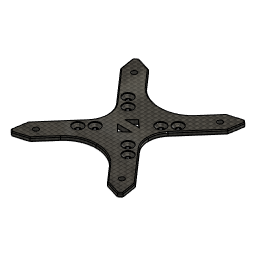
middle_plate (Autodesk Fusion 360 design; units mm, degrees)
Autodesk Fusion 360 part; units mm, degrees
sketch "Sketch1" plane through (0, 0, 0) normal (0, 1, 0) x (1, 0, 0)
  line L0 (25.882765, 29.580303) -> (21.367305, 33.53133) construction
  line L1 (25.882765, 29.580303) -> (30.398225, 25.629275) construction
  line L2 (23.572116, 36.051114) -> (14.916845, 26.159376)
  arc A0 (0, 19.5) -> (14.916845, 26.159376) centre (0.237925, 39.003431) ccw
  line L3 (34.026215, 36.985626) -> (33.083891, 37.81016)
  circle A1 centre (10, 10) radius 1.015
  line L4 (-15, 15) -> (15, 15) construction
  line L5 (-21.367305, 33.53133) -> (7.972627, -0.000021) construction
  line L6 (30.398225, 25.629275) -> (7.972612, 0.000001) construction
  arc A2 (-14.916845, 26.159376) -> (0, 19.5) centre (-0.237925, 39.003431) ccw
  line L7 (21.367305, 33.53133) -> (-7.972627, -0.000021) construction
  line L8 (32.141566, 38.634694) -> (33.083891, 37.81016)
  line L9 (23.572116, 36.051114) -> (32.141566, 38.634694)
  line L10 (-32.141566, 38.634694) -> (-33.083891, 37.81016)
  line L11 (32.603036, 28.149059) -> (34.026215, 36.985626)
  line L12 (0, 0) -> (0, 40.717058) construction
  line L13 (-32.603036, 28.149059) -> (-34.026215, 36.985626)
  line L14 (-10, 10) -> (10, 10) construction
  line L15 (-25.882765, 29.580303) -> (-21.367305, 33.53133) construction
  line L16 (-23.572116, 36.051114) -> (-32.141566, 38.634694)
  line L17 (-23.572116, 36.051114) -> (-14.916845, 26.159376)
  line L18 (-34.026215, 36.985626) -> (-33.083891, 37.81016)
  line L19 (-25.882765, 29.580303) -> (-30.398225, 25.629275) construction
  circle A3 centre (-10, 10) radius 1.015
  line L20 (-0.000752, 6.361835) -> (-4.075325, 2.287262)
  line L21 (4.583143, 2.287262) -> (-0.000752, 6.361835)
  line L22 (0, 0) -> (-12.395289, 0.000003)
  line L23 (-4.075325, 2.287262) -> (4.583143, 2.287262)
  line L24 (-32.603036, 28.149059) -> (-15.606858, 8.724856)
  arc A4 (-12.395289, 0.000003) -> (-15.606858, 8.724856) centre (-25.378902, 0.174315) ccw
  line L25 (32.603036, 28.149059) -> (15.606858, 8.724856)
  arc A5 (15.606858, 8.724856) -> (12.395289, 0.000003) centre (25.378902, 0.174315) ccw
  line L26 (0, 0) -> (50.000001, 0) construction
  arc A6 (0, -19.5) -> (-14.916845, -26.159376) centre (-0.237925, -39.003431) ccw
  line L27 (-15, -15) -> (15, -15) construction
  line L28 (30.398225, -25.629275) -> (7.972612, -0.000001) construction
  line L29 (-32.603036, -28.149059) -> (-15.606858, -8.724856)
  line L30 (32.603036, -28.149059) -> (15.606858, -8.724856)
  arc A7 (12.395289, -0.000003) -> (15.606858, -8.724856) centre (25.378902, -0.174315) ccw
  line L31 (21.367305, -33.53133) -> (-7.972627, 0.000021) construction
  line L32 (-23.572116, -36.051114) -> (-32.141566, -38.634694)
  line L33 (0, 0) -> (-12.395289, -0.000003)
  line L34 (-32.603036, -28.149059) -> (-34.026215, -36.985626)
  circle A8 centre (-10, -10) radius 1.015
  line L35 (-0.000752, -6.361835) -> (-4.075325, -2.287262)
  line L36 (23.572116, -36.051114) -> (14.916845, -26.159376)
  circle A9 centre (10, -10) radius 1.015
  line L37 (-25.882765, -29.580303) -> (-30.398225, -25.629275) construction
  arc A10 (-15.606858, -8.724856) -> (-12.395289, -0.000003) centre (-25.378902, -0.174315) ccw
  line L38 (-21.367305, -33.53133) -> (7.972627, 0.000021) construction
  line L39 (4.583143, -2.287262) -> (-0.000752, -6.361835)
  line L40 (-4.075325, -2.287262) -> (4.583143, -2.287262)
  line L41 (25.882765, -29.580303) -> (21.367305, -33.53133) construction
  line L42 (25.882765, -29.580303) -> (30.398225, -25.629275) construction
  line L43 (-34.026215, -36.985626) -> (-33.083891, -37.81016)
  line L44 (-23.572116, -36.051114) -> (-14.916845, -26.159376)
  line L45 (23.572116, -36.051114) -> (32.141566, -38.634694)
  line L46 (34.026215, -36.985626) -> (33.083891, -37.81016)
  line L47 (32.603036, -28.149059) -> (34.026215, -36.985626)
  line L48 (0, 0) -> (0, -40.717058) construction
  arc A11 (14.916845, -26.159376) -> (0, -19.5) centre (0.237925, -39.003431) ccw
  line L49 (-25.882765, -29.580303) -> (-21.367305, -33.53133) construction
  line L50 (32.141566, -38.634694) -> (33.083891, -37.81016)
  line L51 (-32.141566, -38.634694) -> (-33.083891, -37.81016)
  line L52 (-10, -10) -> (10, -10) construction
  circle A12 centre (-26.106671, -29.832074) radius 1.525
  circle A13 centre (-19.710816, -22.523297) radius 1.525
  line L53 (-25.88455, -29.578249) -> (-30.399804, -25.626985) construction
  line L54 (-25.88455, -29.578249) -> (-21.369297, -33.529512) construction
  circle A14 centre (-19.710816, 22.523297) radius 1.525
  circle A15 centre (-26.106671, 29.832074) radius 1.525
  circle A16 centre (19.710816, 22.523297) radius 1.525
  circle A17 centre (26.106671, 29.832074) radius 1.525
  circle A18 centre (19.710816, -22.523297) radius 1.525
  circle A19 centre (26.106671, -29.832074) radius 1.525
  circle A20 centre (0, 0) radius 6.361835
  line L55 (15.25, 15.25) -> (-15.25, 15.25) construction
  line L56 (-15.25, 15.25) -> (-15.25, -15.25) construction
  line L57 (-15.25, -15.25) -> (15.25, -15.25) construction
  line L58 (15.25, -15.25) -> (15.25, 15.25) construction
  line L59 (15.25, 15.25) -> (-15.25, -15.25) construction
  line L60 (-15.25, 15.25) -> (15.25, -15.25) construction
  circle A21 centre (15.25, 15.25) radius 1.525
  circle A22 centre (-15.25, 15.25) radius 1.525
  circle A23 centre (-15.25, -15.25) radius 1.525
  circle A24 centre (15.25, -15.25) radius 1.525
  point P0 (15, 15)
  point P1 (10, 10)
  point P2 (0, 17.5)
  point P3 (0, 40.717058)
  point P4 (-7.972609, 0)
  point P5 (7.972609, 0)
  point P6 (-7.972609, 0)
  point P7 (7.972609, 0)
  point P8 (0, -40.717058)
  point P9 (-7.972609, 0)
  point P10 (-7.972609, 0)
  point P11 (0, -17.5)
  point P12 (7.972609, 0)
  point P13 (7.972609, 0)
  point P14 (10, -10)
  point P15 (15, -15)
  point P16 (15.25, 15.25)
  dimension "d3" = 30
  dimension "d5" = 20
  dimension "d42" = 2.03
  dimension "d90" = 6
  dimension "d91" = 6
  dimension "d75" = 30.5
  dimension "d76" = 30.5
  dimension "d77" = 3.05
  dimension "d78" = 3.05
  dimension "d79" = 3.05
  dimension "d80" = 3.05
  constraint coincident L12.start L22.start
  constraint coincident L14.start A3.centre
  constraint perpendicular L5 L15
  constraint symmetric L22.start L26.start L12
  constraint tangent L5 A2
  constraint coincident A0.start L12
  constraint symmetric A0.start A2.end L12
  constraint symmetric A0 A2 L12
  constraint symmetric L12 A4 A5
  constraint perpendicular L12 L26
  constraint symmetric L12.start L26 L22.start
  constraint symmetric P0 L26 P15
  constraint symmetric P1 L26 P14
  constraint symmetric P2 L26 P11
  constraint symmetric A0.start L26 A6.start
  constraint symmetric L4.start L26 L27.start
  constraint symmetric L14.start L26 A8.centre
  constraint symmetric A0 L26 A11
  constraint symmetric A1 L26 A9
  constraint symmetric A2 L26 A6
  constraint symmetric A3 L26 A8
  constraint symmetric A4 L26 A10
  constraint symmetric A5 L26 A7
  constraint symmetric L26 A12 A15
  constraint symmetric L26 A13 A14
  constraint symmetric L12 A12 A19
  constraint symmetric L12 A13 A18
  constraint symmetric L12 A14 A16
  constraint symmetric L12 A15 A17
  constraint horizontal L55
  constraint perpendicular L55 L56
  constraint parallel L55 L57
  constraint parallel L56 L58
  constraint coincident L59 L12.start
  constraint coincident L60 L12.start
  constraint coincident P16 L55.start
  constraint coincident L55.end L56.start
  constraint coincident L56.end L57.start
  constraint coincident L57.end L58.start
  measures "d3" distance of P0 L4.start
  measures "d5" distance of P1 L14.start
  measures "d42" diameter of A3
  measures "d75" distance of L56.end L57.end
  measures "d76" distance of L55.end L56.end
  measures "d77" diameter of A21
  measures "d78" diameter of A22
  measures "d79" diameter of A23
  measures "d80" diameter of A24
extrude "Extrude1" add sketch "Sketch1" along normal blind 2.5 contours L2 A0 L3 A2 L8 L9 L10 L11 L13 L16 L17 L18 L24 A4 L25 A5 A6 L29 L30 A7 L32 L34 L36 A10 L43 L44 L45 L46 L47 A11 L50 L51 | A20 | A13 | A14 | A16 | A18 | A21 | A22 | A23 | A24 picked at (-4.25837, 12.121682) picked at (-1.189169, 0.762421) picked at (-19.310424, -22.106819) picked at (-19.310424, 22.939775) picked at (20.111208, 22.939775) picked at (19.365938, -22.798328) picked at (15.584647, 15.088843) picked at (-15.092222, 14.609617) picked at (-15.663329, -15.174237) picked at (15.539984, -15.114837)
ref_plane "WorkPlane1" through (0, 2, 0) normal (0, 1, 0) x (1, 0, 0)
sketch "Sketch2" plane through (0, 2, 0) normal (0, 1, 0) x (-1, 0, 0)
  circle A0 centre (-19.710816, 22.523297) radius 1.525
  circle A1 centre (-26.106671, 29.832074) radius 1.525
  circle A2 centre (-10, -10) radius 1.015
  circle A3 centre (19.710816, 22.523297) radius 1.525
  circle A4 centre (-10, 10) radius 1.015
  line L0 (-4.583143, -2.287262) -> (4.075325, -2.287262)
  line L1 (4.075325, -2.287262) -> (0.000752, -6.361835)
  line L2 (0.000752, -6.361835) -> (-4.583143, -2.287262)
  circle A5 centre (-26.106671, -29.832074) radius 1.525
  circle A6 centre (19.710816, -22.523297) radius 1.525
  circle A7 centre (10, 10) radius 1.015
  circle A8 centre (10, -10) radius 1.015
  line L3 (0.000752, 6.361835) -> (4.075325, 2.287262)
  line L4 (4.075325, 2.287262) -> (-4.583143, 2.287262)
  line L5 (-4.583143, 2.287262) -> (0.000752, 6.361835)
  circle A9 centre (26.106671, 29.832074) radius 1.525
  circle A10 centre (-19.710816, -22.523297) radius 1.525
  circle A11 centre (26.106671, -29.832074) radius 1.525
  line L6 (23.572116, 36.051114) -> (14.916845, 26.159376)
  arc A12 (0, 19.5) -> (14.916845, 26.159376) centre (0.237925, 39.003431) ccw
  arc A13 (-14.916845, 26.159376) -> (0, 19.5) centre (-0.237925, 39.003431) ccw
  line L7 (-14.916845, 26.159376) -> (-23.572116, 36.051114)
  line L8 (-23.572116, 36.051114) -> (-32.141566, 38.634694)
  line L9 (-32.141566, 38.634694) -> (-34.026215, 36.985626)
  line L10 (-34.026215, 36.985626) -> (-32.603036, 28.149059)
  line L11 (-32.603036, 28.149059) -> (-15.606858, 8.724856)
  arc A14 (-12.395289, 0.000003) -> (-15.606858, 8.724856) centre (-25.378902, 0.174315) ccw
  arc A15 (-15.606858, -8.724856) -> (-12.395289, -0.000003) centre (-25.378902, -0.174315) ccw
  line L12 (-15.606858, -8.724856) -> (-32.603036, -28.149059)
  line L13 (-32.603036, -28.149059) -> (-34.026215, -36.985626)
  line L14 (-34.026215, -36.985626) -> (-32.141566, -38.634694)
  line L15 (-32.141566, -38.634694) -> (-23.572116, -36.051114)
  line L16 (-23.572116, -36.051114) -> (-14.916845, -26.159376)
  arc A16 (0, -19.5) -> (-14.916845, -26.159376) centre (-0.237925, -39.003431) ccw
  arc A17 (14.916845, -26.159376) -> (0, -19.5) centre (0.237925, -39.003431) ccw
  line L17 (14.916845, -26.159376) -> (23.572116, -36.051114)
  line L18 (23.572116, -36.051114) -> (32.141566, -38.634694)
  line L19 (32.141566, -38.634694) -> (34.026215, -36.985626)
  line L20 (34.026215, -36.985626) -> (32.603036, -28.149059)
  line L21 (32.603036, -28.149059) -> (15.606858, -8.724856)
  arc A18 (12.395289, -0.000003) -> (15.606858, -8.724856) centre (25.378902, -0.174315) ccw
  arc A19 (15.606858, 8.724856) -> (12.395289, 0.000003) centre (25.378902, 0.174315) ccw
  line L22 (15.606858, 8.724856) -> (32.603036, 28.149059)
  line L23 (32.603036, 28.149059) -> (34.026215, 36.985626)
  line L24 (34.026215, 36.985626) -> (32.141566, 38.634694)
  line L25 (32.141566, 38.634694) -> (23.572116, 36.051114)
  circle A20 centre (-15.25, -15.25) radius 1.525
  circle A21 centre (15.25, -15.25) radius 1.525
  circle A22 centre (15.25, 15.25) radius 1.525
  circle A23 centre (-15.25, 15.25) radius 1.525
  dimension "d81" = 3.05
  dimension "d82" = 3.05
  dimension "d83" = 3.05
  dimension "d84" = 3.05
  measures "d81" diameter of A22
  measures "d82" diameter of A23
  measures "d83" diameter of A20
  measures "d84" diameter of A21
hole "Hole1" at (-15.25, 2, 15.25) at (-15.25, 2, -15.25) at (15.25, 2, -15.25) at (15.25, 2, 15.25) at (10, 2, 10) at (10, 2, -10) at (-10, 2, -10) at (-10, 2, 10) direction (0, -1, 0) diameter 3.2 depth 8 tip angle 118 countersink diameter 6.2 countersink angle 90
hole "Hole2" at (-10, 2, 10) at (-10, 2, -10) at (10, 2, -10) at (10, 2, 10) direction (0, -1, 0) diameter 3.2 depth 8 tip angle 118 countersink diameter 6.2 countersink angle 90
sketch "Sketch3" plane through (0, 2.5, 0) normal (0, 1, 0) x (-1, 0, 0)
  circle A0 centre (26.106671, -29.832074) radius 1.525
  circle A1 centre (26.106671, 29.832074) radius 1.525
  line L0 (0.000752, 6.361835) -> (4.075325, 2.287262)
  line L1 (4.075325, 2.287262) -> (-4.583143, 2.287262)
  line L2 (-4.583143, 2.287262) -> (0.000752, 6.361835)
  circle A2 centre (-26.106671, 29.832074) radius 1.525
  circle A3 centre (-26.106671, -29.832074) radius 1.525
  line L3 (-4.583143, -2.287262) -> (4.075325, -2.287262)
  line L4 (4.075325, -2.287262) -> (0.000752, -6.361835)
  line L5 (0.000752, -6.361835) -> (-4.583143, -2.287262)
  line L6 (23.572116, 36.051114) -> (14.916845, 26.159376)
  arc A4 (0, 19.5) -> (14.916845, 26.159376) centre (0.237925, 39.003431) ccw
  arc A5 (-14.916845, 26.159376) -> (0, 19.5) centre (-0.237925, 39.003431) ccw
  line L7 (-14.916845, 26.159376) -> (-23.572116, 36.051114)
  line L8 (-23.572116, 36.051114) -> (-32.141566, 38.634694)
  line L9 (-32.141566, 38.634694) -> (-34.026215, 36.985626)
  line L10 (-34.026215, 36.985626) -> (-32.603036, 28.149059)
  line L11 (-32.603036, 28.149059) -> (-15.606858, 8.724856)
  arc A6 (-12.395289, 0.000003) -> (-15.606858, 8.724856) centre (-25.378902, 0.174315) ccw
  arc A7 (-15.606858, -8.724856) -> (-12.395289, -0.000003) centre (-25.378902, -0.174315) ccw
  line L12 (-15.606858, -8.724856) -> (-32.603036, -28.149059)
  line L13 (-32.603036, -28.149059) -> (-34.026215, -36.985626)
  line L14 (-34.026215, -36.985626) -> (-32.141566, -38.634694)
  line L15 (-32.141566, -38.634694) -> (-23.572116, -36.051114)
  line L16 (-23.572116, -36.051114) -> (-14.916845, -26.159376)
  arc A8 (0, -19.5) -> (-14.916845, -26.159376) centre (-0.237925, -39.003431) ccw
  arc A9 (14.916845, -26.159376) -> (0, -19.5) centre (0.237925, -39.003431) ccw
  line L17 (14.916845, -26.159376) -> (23.572116, -36.051114)
  line L18 (23.572116, -36.051114) -> (32.141566, -38.634694)
  line L19 (32.141566, -38.634694) -> (34.026215, -36.985626)
  line L20 (34.026215, -36.985626) -> (32.603036, -28.149059)
  line L21 (32.603036, -28.149059) -> (15.606858, -8.724856)
  arc A10 (12.395289, -0.000003) -> (15.606858, -8.724856) centre (25.378902, -0.174315) ccw
  arc A11 (15.606858, 8.724856) -> (12.395289, 0.000003) centre (25.378902, 0.174315) ccw
  line L22 (15.606858, 8.724856) -> (32.603036, 28.149059)
  line L23 (32.603036, 28.149059) -> (34.026215, 36.985626)
  line L24 (34.026215, 36.985626) -> (32.141566, 38.634694)
  line L25 (32.141566, 38.634694) -> (23.572116, 36.051114)
  circle A12 centre (-10, -10) radius 1.015
  circle A13 centre (-10, 10) radius 1.015
  circle A14 centre (10, 10) radius 1.015
  circle A15 centre (10, -10) radius 1.015
sketch "Sketch5" plane through (0, 2, 0) normal (0, -1, 0) x (1, 0, 0)
  circle A0 centre (15.25, 15.25) radius 3.1
  circle A1 centre (15.25, -15.25) radius 3.1
  circle A2 centre (-15.25, 15.25) radius 3.1
  circle A3 centre (-15.25, -15.25) radius 3.1
  circle A4 centre (15.25, 15.25) radius 3.1
  line L0 (-0.000752, 6.361835) -> (4.583143, 2.287262)
  line L1 (4.583143, 2.287262) -> (-4.075325, 2.287262)
  line L2 (-4.075325, 2.287262) -> (-0.000752, 6.361835)
  circle A5 centre (-26.106671, -29.832074) radius 1.525
  circle A6 centre (26.106671, -29.832074) radius 1.525
  line L3 (4.583143, -2.287262) -> (-0.000752, -6.361835)
  line L4 (-0.000752, -6.361835) -> (-4.075325, -2.287262)
  line L5 (-4.075325, -2.287262) -> (4.583143, -2.287262)
  circle A7 centre (26.106671, 29.832074) radius 1.525
  circle A8 centre (-26.106671, 29.832074) radius 1.525
  arc A9 (-12.395289, -0.000003) -> (-15.606858, -8.724856) centre (-25.378902, -0.174315) cw
  line L6 (-15.606858, -8.724856) -> (-32.603036, -28.149059)
  line L7 (-32.603036, -28.149059) -> (-34.026215, -36.985626)
  line L8 (-34.026215, -36.985626) -> (-32.141566, -38.634694)
  line L9 (-32.141566, -38.634694) -> (-23.572116, -36.051114)
  line L10 (-23.572116, -36.051114) -> (-14.916845, -26.159376)
  arc A10 (-14.916845, -26.159376) -> (0, -19.5) centre (-0.237925, -39.003431) cw
  arc A11 (0, -19.5) -> (14.916845, -26.159376) centre (0.237925, -39.003431) cw
  line L11 (14.916845, -26.159376) -> (23.572116, -36.051114)
  line L12 (23.572116, -36.051114) -> (32.141566, -38.634694)
  line L13 (32.141566, -38.634694) -> (34.026215, -36.985626)
  line L14 (34.026215, -36.985626) -> (32.603036, -28.149059)
  line L15 (32.603036, -28.149059) -> (15.606858, -8.724856)
  arc A12 (15.606858, -8.724856) -> (12.395289, -0.000003) centre (25.378902, -0.174315) cw
  arc A13 (12.395289, -0.000003) -> (15.606858, 8.724856) centre (25.378902, 0.174315) cw
  line L16 (15.606858, 8.724856) -> (32.603036, 28.149059)
  line L17 (32.603036, 28.149059) -> (34.026215, 36.985626)
  line L18 (34.026215, 36.985626) -> (32.141566, 38.634694)
  line L19 (32.141566, 38.634694) -> (23.572116, 36.051114)
  line L20 (23.572116, 36.051114) -> (14.916845, 26.159376)
  arc A14 (14.916845, 26.159376) -> (0, 19.5) centre (0.237925, 39.003431) cw
  arc A15 (0, 19.5) -> (-14.916845, 26.159376) centre (-0.237925, 39.003431) cw
  line L21 (-14.916845, 26.159376) -> (-23.572116, 36.051114)
  line L22 (-23.572116, 36.051114) -> (-32.141566, 38.634694)
  line L23 (-32.141566, 38.634694) -> (-34.026215, 36.985626)
  line L24 (-34.026215, 36.985626) -> (-32.603036, 28.149059)
  line L25 (-32.603036, 28.149059) -> (-15.606858, 8.724856)
  arc A16 (-15.606858, 8.724856) -> (-12.395289, -0.000003) centre (-25.378902, 0.174315) cw
  circle A17 centre (-10, -10) radius 3.1
  circle A18 centre (10, 10) radius 3.1
  circle A19 centre (10, -10) radius 3.1
  circle A20 centre (-10, 10) radius 3.1
  circle A21 centre (-10, -10) radius 1.015
  circle A22 centre (-10, 10) radius 1.015
  circle A23 centre (10, 10) radius 1.015
  circle A24 centre (10, -10) radius 1.015
extrude "Extrude3" cut sketch "Sketch5" against normal blind 6.222 contours A0 A4 | A1 | A2 | A3 | A17 | A18 | A19 | A20 picked at (16.271792, 16.809701) picked at (14.480972, -14.393144) picked at (-14.492513, 15.952845) picked at (-16.445306, -14.841491) picked at (-7.61032, -10.204436) picked at (12.38968, 9.795564) picked at (12.38968, -10.204436) picked at (-7.61032, 9.795564)
chamfer "Chamfer1" distance 0.5 angle 45 56 edges at (-19.24448, 2.5, -31.105245) (-8.189177, 2.5, -21.192816) (8.189177, 2.5, -21.192816) (19.24448, 2.5, -31.105245) (27.856841, 2.5, -37.342904) (33.08389, 2.5, -37.81016) (33.314625, 2.5, -32.567343) (24.104947, 2.5, -18.436957) (13.193429, 2.5, -4.659718) (13.193429, 2.5, 4.659718) (24.104947, 2.5, 18.436957) (33.314625, 2.5, 32.567343) (33.08389, 2.5, 37.81016) (27.856841, 2.5, 37.342904) (19.24448, 2.5, 31.105245) (8.189177, 2.5, 21.192816) (-8.189177, 2.5, 21.192816) (-19.24448, 2.5, 31.105245) (-27.856841, 2.5, 37.342904) (-33.08389, 2.5, 37.81016) (-33.314625, 2.5, 32.567343) (-24.104947, 2.5, 18.436957) (-13.193429, 2.5, 4.659718) (-13.193429, 2.5, -4.659718) (-24.104947, 2.5, -18.436957) (-33.314625, 2.5, -32.567343) (-33.08389, 2.5, -37.81016) (-27.856841, 2.5, -37.342904) (-8.189177, 0, -21.192816) (-19.24448, 0, -31.105245) (8.189177, 0, -21.192816) (19.24448, 0, -31.105245) (27.856841, 0, -37.342904) (33.08389, 0, -37.81016) (33.314625, 0, -32.567343) (24.104947, 0, -18.436957) (13.193429, 0, -4.659718) (13.193429, 0, 4.659718) (24.104947, 0, 18.436957) (33.314625, 0, 32.567343) (33.08389, 0, 37.81016) (27.856841, 0, 37.342904) (19.24448, 0, 31.105245) (8.189177, 0, 21.192816) (-8.189177, 0, 21.192816) (-19.24448, 0, 31.105245) (-27.856841, 0, 37.342904) (-33.08389, 0, 37.81016) (-33.314625, 0, 32.567343) (-24.104947, 0, 18.436957) (-13.193429, 0, 4.659718) (-13.193429, 0, -4.659718) (-24.104947, 0, -18.436957) (-33.314625, 0, -32.567343) (-33.08389, 0, -37.81016) (-27.856841, 0, -37.342904)
